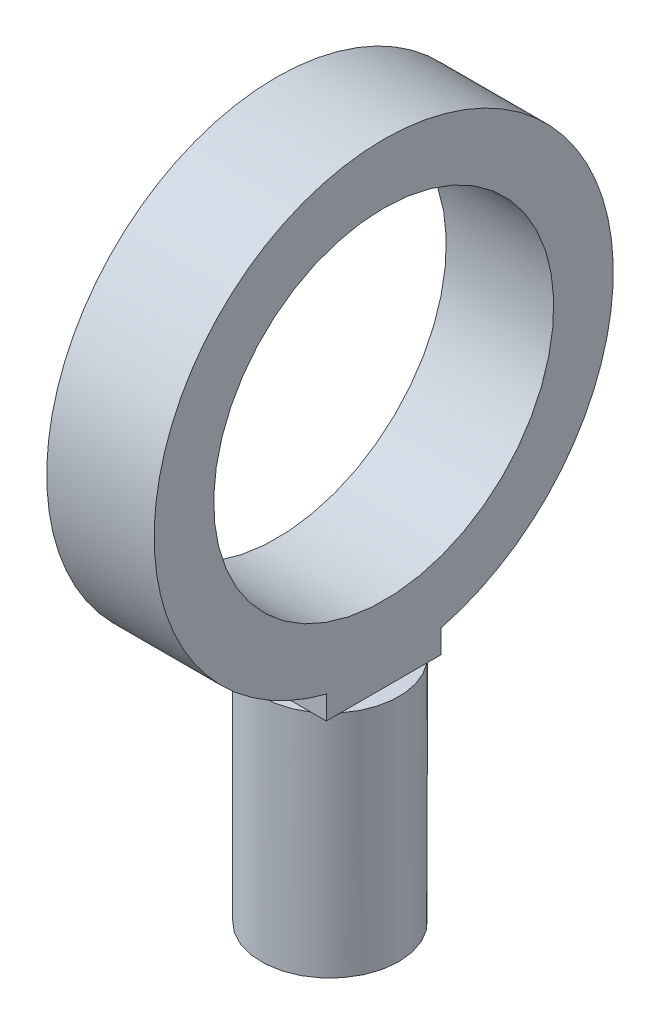
# Autodesk Inventor part: M12 Eye Bolt
Saved by Autodesk Inventor 2019.4 (Build 234330000, 330)
## iProperties
Created: 2020-02-01
Part Number: M12 Eye Bolt
Material: Steel, Alloy
Document SubType Name: Modeling
Designer: Mark
Mass: 26.9359 g
Surface Area: 26.3093 cm^2
Volume: 3.48459 cm^3
Density: 7.73 g/cm^3
Appearance: Semi-Polished
Author: Mark
Autodesk Inventor part; units mm, degrees
ref_plane "YZ Plane" through (0, 0, 0) normal (1, 0, 0) x (0, 1, 0)
ref_plane "XZ Plane" through (0, 0, 0) normal (0, 1, 0) x (-1, 0, 0)
ref_plane "XY Plane" through (0, 0, 0) normal (0, 0, 1) x (1, 0, 0)
sketch "Sketch1" plane through (0, 0.5, 0) normal (1, 0, 0) x (0, 1, 0)
  circle A0 centre (7.8907, 0) radius 14.815
  arc A1 (-11.5, -4.899) -> (-11.5, 4.899) centre (7.8907, 0) ccw
  line L0 (-13.5, 5) -> (-11.5, 5)
  line L1 (-11.5, 5) -> (-11.5, -5)
  line L2 (-11.5, -5) -> (-13.5, -5)
  line L3 (-13.5, -5) -> (-13.5, 5)
  line L4 (-13.5, 5) -> (-11.5, -5) construction
  line L5 (-11.5, 5) -> (-13.5, -5) construction
  dimension "d3" = 29.63
  dimension "d2" = 40
  dimension "d0" = 2
  dimension "d1" = 10
  constraints: 12 end point, 2 centre point, 2 coincident, 2 parallel, 2 point on circle, 2 point on line, 1 horizontal, 1 perpendicular
  measures "d3" diameter of A0
  measures "d2" diameter of A1
  measures "d0" distance of L1.end L2.end
  measures "d1" distance of L0.end L1.end
extrude "Extrusion1" add sketch "Sketch1" along normal blind 9.36
sketch "Sketch2" plane through (0, -13, -5) normal (0, -1, 0) x (1, 0, 0)
  circle A0 centre (4.68, 5) radius 6
  line L0 (9.36, 10) -> (9.36, 0) projected
  line L1 (0, 0) -> (9.36, 0) projected
  point P0 (0, 5)
  dimension "d7" = 12
  dimension "d9" = 4.68
  dimension "d8" = 5
  constraints: 1 centre point
  measures "d7" diameter of A0
  measures "d9" distance from line of L0 A0.centre
  measures "d8" distance from line of L1 A0.centre
extrude "Extrusion2" add sketch "Sketch2" along normal blind 20 contours A0 L0 | L0 A0 L1 | L1 A0 picked at (6.0374, 4.0549)
body "Solid1"
